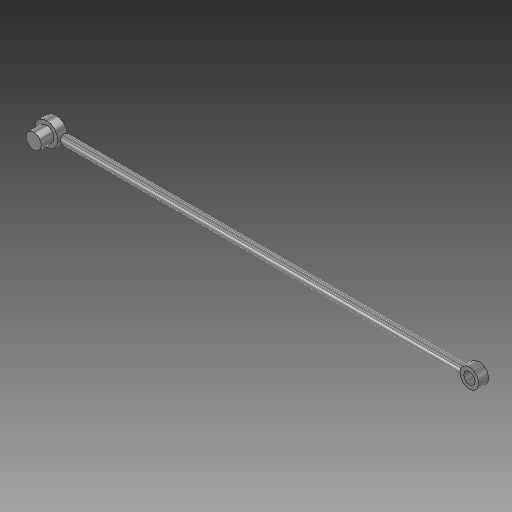
# Autodesk Inventor part: 101-04
Saved by Autodesk Inventor 2019 (Build 230136000, 136)
## iProperties
Company: Autodesk Inc.
Created: 2017-03-14
Part Number: 101-04
Material: Aluminum 6061
Document SubType Name: Modeling
Designer: Autodesk Inc.
Density: 2.7 g/cm^3
Appearance: Aluminum - Anodized Glossy (Grey)
Mass: 1.57173 g
Surface Area: 9.92634 cm^2
Volume: 0.582123 cm^3
Author: Inventor
Autodesk Inventor part; units mm, degrees
ref_plane "YZ Plane" through (0, 0, 0) normal (1, 0, 0) x (0, 1, 0)
ref_plane "XZ Plane" through (0, 0, 0) normal (0, 1, 0) x (-1, 0, 0)
ref_plane "XY Plane" through (0, 0, 0) normal (0, 0, 1) x (1, 0, 0)
sketch "Sketch1" plane through (0, 0, 0) normal (1, 0, 0) x (0, 1, 0)
  circle A0 centre (0, 0) radius 1.15
  dimension "d0" = 2.3
  constraints: 1 centre point, 1 coincident
  measures "d0" diameter of A0
extrude "Extrusion1" add sketch "Sketch1" along normal blind 105
sketch "Sketch3" plane through (0, 0, 0) normal (0, 1, 0) x (-1, 0, 0)
  line L0 (-105.5, 1.25) -> (-105.5, -1.25)
  line L1 (-107, 4.3664) -> (-107, -6.1894)
  line L2 (-105, 1.15) -> (-105, -1.15) projected
  line L3 (-105.5, 1.25) -> (-104.5, 1.25)
  line L4 (-104.5, 1.25) -> (-104.5, -1.25)
  line L5 (-104.5, -1.25) -> (-105.5, -1.25)
  point P0 (0, 0)
  dimension "d7" = 2.5
  dimension "d10" = 1
  dimension "d11" = 0.5
  dimension "d12" = 2.5
  constraints: 10 end point, 2 horizontal, 2 vertical, 1 parallel, 1 perpendicular
  measures "d7" distance of L0.start L0.end
  measures "d10" distance of L4.end L0.end
  measures "d11" distance between parallel lines of L4 L2
  measures "d12" distance between parallel lines of L1 L4
revolve "Revolution1" add sketch "Sketch3" angle 360 about axis through (107, 0, 4.3664) along (0, 0, -1)
sketch "Sketch4" plane through (0, 0, 0) normal (0, 1, 0) x (-1, 0, 0)
  line L0 (-2.6081, 0) -> (2.6081, 0)
  line L1 (0.5, 0) -> (0.5, 1.25)
  line L2 (0, -1.15) -> (0, 1.15) projected
  line L3 (0.5, 1.25) -> (3.5, 1.25)
  line L4 (3.5, -1.25) -> (0.5, -1.25)
  line L5 (0.5, -1.25) -> (0.5, 0)
  line L6 (3.5, 1.25) -> (3.5, -1.25)
  point P0 (0, 0)
  point P1 (0, 0)
  dimension "d14" = 0.5
  dimension "d18" = 3
  constraints: 12 end point, 4 horizontal, 2 equal length, 2 vertical, 1 coincident, 1 midpoint, 1 point on line
  measures "d14" distance between parallel lines of L2 L1
  measures "d18" distance between parallel lines of L5 L6
revolve "Revolution2" add sketch "Sketch4" angle 360 about axis through (-3.5, 0, 1.25) along (0, 0, -1)
sketch "Sketch5" plane through (-3.5, 0, 1.25) normal (0, 0, 1) x (1, 0, 0)
  circle A0 centre (0, 0) radius 3 projected
  circle A1 centre (0, 0) radius 2
  point P0 (3.5, 0)
  dimension "d20" = 4
  constraints: 1 centre point, 1 coincident
  measures "d20" diameter of A1
extrude "Extrusion2" add sketch "Sketch5" along normal blind 3.3 contours A1
sketch "Sketch6" plane through (-3.5, 0, -1.25) normal (0, 0, -1) x (-1, 0, 0)
  circle A0 centre (0, 0) radius 2 projected
  point P0 (-3.5, 0)
extrude "Extrusion3" add sketch "Sketch6" along normal blind 0.3
body "Solid1"
